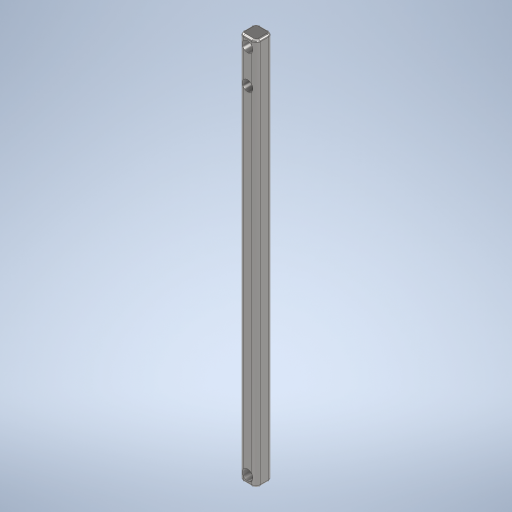
# Autodesk Inventor part: cata pult
Saved by Autodesk Inventor 2023 (Build 270158000, 158)
## iProperties
Created: 2022-07-10
Part Number: cata pult
Material: Stainless Steel
Document SubType Name: Modeling
Designer: aaron
Density: 8 g/cm^3
Appearance: Semi-Polished
Author: aaron
Autodesk Inventor part; units mm, degrees
ref_plane "YZ Plane" through (0, 0, 0) normal (1, 0, 0) x (0, 1, 0)
ref_plane "XZ Plane" through (0, 0, 0) normal (0, 1, 0) x (-1, 0, 0)
ref_plane "XY Plane" through (0, 0, 0) normal (0, 0, 1) x (1, 0, 0)
sketch "Sketch1" plane through (0, 0, 0) normal (0, 1, 0) x (-1, 0, 0)
  point P0 (0, 0)
sketch "Sketch2" plane through (0, 0, 0) normal (0, 1, 0) x (-1, 0, 0)
  line L0 (-3.175, -3.175) -> (3.175, -3.175)
  line L1 (3.175, -3.175) -> (3.175, 3.175)
  line L2 (3.175, 3.175) -> (-3.175, 3.175)
  line L3 (-3.175, 3.175) -> (-3.175, -3.175)
  line L4 (-3.175, -3.175) -> (3.175, 3.175) construction
  line L5 (3.175, -3.175) -> (-3.175, 3.175) construction
  point P0 (0, 0)
  dimension "d0" = 6.35
  dimension "d1" = 6.35
  constraints: 12 end point, 2 midpoint, 2 parallel, 1 horizontal, 1 perpendicular
  measures "d0" distance of L2.end L1.end
  measures "d1" distance of L1.end L0.end
extrude "Extrusion1" add sketch "Sketch2" along normal blind 146.05
sketch "Sketch3" plane through (-3.175, 0, 3.175) normal (0, 0, 1) x (1, 0, 0)
  circle A0 centre (3.175, 3.175) radius 1.9844
  line L0 (0, 0) -> (6.35, 0) projected
  line L1 (6.35, 0) -> (6.35, 146.05) projected
  point P0 (3.175, 0)
  dimension "d4" = 3.9688
  dimension "d5" = 3.175
  dimension "d6" = 3.175
  constraints: 1 centre point
  measures "d4" diameter of A0
  measures "d5" distance from line of L0 A0.centre
  measures "d6" distance from line of L1 A0.centre
extrude "Extrusion2" cut sketch "Sketch3" against normal blind 292.1
sketch "Sketch4" plane through (-3.175, 0, 3.175) normal (0, 0, 1) x (1, 0, 0)
  circle A0 centre (3.175, 142.875) radius 1.9844
  circle A1 centre (3.175, 130.175) radius 1.9844
  line L0 (6.35, 0) -> (6.35, 146.05) projected
  line L1 (0, 0) -> (0, 146.05) projected
  circle A2 centre (3.175, 3.175) radius 1.9844 projected
  point P0 (3.175, 0)
  dimension "d9" = 3.9688
  dimension "d10" = 3.9688
  dimension "d11" = 12.7
  dimension "d12" = 3.175
  dimension "d13" = 3.175
  dimension "d14" = 127
  constraints: 2 centre point
  measures "d9" diameter of A0
  measures "d10" diameter of A1
  measures "d11" distance of A0.centre A1.centre
  measures "d12" distance from line of L0 A0.centre
  measures "d13" distance from line of L1 A1.centre
  measures "d14" distance of A2.centre A1.centre
extrude "Extrusion3" cut sketch "Sketch4" against normal blind 292.1 contours A0 | A1
fillet "Fillet1" radius 1.5875 4 edges at (3.175, 73.025, 3.175) (3.175, 73.025, -3.175) (-3.175, 73.025, -3.175) (-3.175, 73.025, 3.175)
fillet "Fillet2" radius 0.7937 16 edges at (2.71, 146.05, -2.71) (0, 146.05, -3.175) (-2.71, 146.05, -2.71) (-3.175, 146.05, 0) (-2.71, 146.05, 2.71) (0, 146.05, 3.175) (2.71, 146.05, 2.71) (3.175, 146.05, 0) (2.71, 0, -2.71) (0, 0, -3.175) (-2.71, 0, -2.71) (-3.175, 0, 0) (-2.71, 0, 2.71) (0, 0, 3.175) (2.71, 0, 2.71) (3.175, 0, 0)
body "Solid1"
